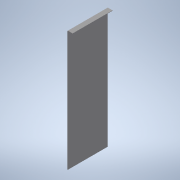
# Autodesk Inventor part: LeftWall
Saved by Autodesk Inventor 2020 (Build 240168000, 168)
## iProperties
Created: 2025-10-20
Part Number: LeftWall
Material: Carbon Steel - A36
Document SubType Name: Sheet Metal
Designer: pcajigal
Density: 7.86 g/cm^3
Sheet Metal Rule: 1/4 Steel
Sheet Metal Width: 0.000 in
Sheet Metal Length: 0.000 in
Sheet Metal Area: 0.000 in^2
Appearance: Steel
Author: pcajigal
Autodesk Inventor part; units mm, degrees
ref_plane "YZ Plane" through (0, 0, 0) normal (1, 0, 0) x (0, 1, 0)
ref_plane "XZ Plane" through (0, 0, 0) normal (0, 1, 0) x (-1, 0, 0)
ref_plane "XY Plane" through (0, 0, 0) normal (0, 0, 1) x (1, 0, 0)
sketch "Sketch28" plane through (0, 0, 0) normal (1, 0, 0) x (0, 1, 0)
  line L0 (0, 0) -> (2336.8, 0)
  line L1 (2336.8, 0) -> (2336.8, 774.7)
  line L2 (2336.8, 774.7) -> (0, 774.7)
  line L3 (0, 774.7) -> (0, 0)
  dimension "LARGO" = 774.7
  dimension "ALTO" = 2336.8
  measures "LARGO" distance of L0.end L1.end
  measures "ALTO" distance of L1.end L2.end
extrude "Plate26" add sketch "Sketch28" along normal blind 6.35
sketch "Sketch29" plane through (0, 2330.45, 774.7) normal (0, 1, 0) x (-1, 0, 0)
  line L0 (0, -774.7) -> (0, 0)
  line L1 (0, 0) -> (-101.6, 0)
  line L2 (-101.6, 0) -> (-101.6, -774.7)
  line L3 (-101.6, -774.7) -> (0, -774.7)
  constraints: 6 end point, 1 horizontal, 1 perpendicular, 1 vertical
edge flange "Flange23" height 101.6 angle 90 thickness 6.35 bend radius 6.35 thickness toward (0, 1, 0) relief straight relief width 6.35 relief depth 3.175 edges at (6.35, 2336.8, 387.35) wall of the first edge with corners at (0, 2330.45, 0) (0, 2330.45, 774.7) (101.6, 2330.45, 774.7) (101.6, 2330.45, 0)
bend "Bend23"
corner "Corner22"
equation "\"d228\" = Thickness"
equation "\"d229\" = BendReliefWidth"
equation "\"d230\" = BendReliefDepth"
equation "\"d231\" = MinimumRemnant"
equation "\"d232\" = TransitionRadius"
equation "\"d235\" = BendRadius"
equation "\"d236\" = CornerReliefSize"
equation "\"d237\" = GapSize"
equation "\"d238\" = JacobiRadiusSize"
equation "\"BendRadius\" = Thickness"
equation "\"BendReliefWidth\" = Thickness"
equation "\"BendReliefDepth\" = 0.5 * Thickness"
equation "\"CornerReliefSize\" = 4 * Thickness"
equation "\"MinimumRemnant\" = 2 * Thickness"
equation "\"TransitionRadius\" = BendRadius"
equation "\"d2\" = BendRadius"
equation "\"JacobiRadiusSize\" = BendRadius"
equation "\"GapSize\" = Thickness"
equation "\"d12\" = BendRadius"
equation "\"d215\" = BendRadius"
equation "\"Thickness\" = 6.35"
body "Solid3"
